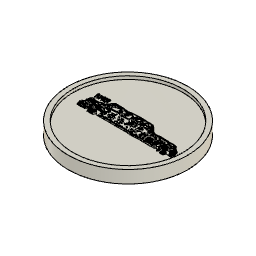
Pink Limo Cup Holder v2 (Autodesk Fusion 360 design; units mm, degrees)
Autodesk Fusion 360 part; units mm, degrees
(part 1 of 5)
sketch "Sketch1" plane through (0, 0, 0) normal (0, 0, 1) x (1, 0, 0)
  circle A0 centre (0, 0) radius 35
  circle A1 centre (0, 0) radius 38
  dimension "d1" = 70
  dimension "d2" = 3
  constraint coincident A0.centre A1.centre
  measures "d1" diameter of A0
extrude "Extrude1" add sketch "Sketch1" along normal blind 8
sketch "Sketch2" plane through (0, 0, 0) normal (0, 0, 1) x (1, 0, 0)
extrude "Extrude2" add sketch "Sketch1" along normal blind 4 contours A0
sketch "Sketch3" plane through (0, 0, 4) normal (0, 0, 1) x (-1, 0, 0)
  circle A0 centre (0, 0) radius 35
  spline S0 degree 3 poles (19.6297, -8.0291) (19.7741, -7.993) (19.7921, -7.8305) (19.7921, -6.2782) knots 0 0 0 0 1 1 1 1
  spline S1 degree 3 poles (19.7921, -6.2782) (19.7921, -5.0869) (19.765, -4.5815) (19.6928, -4.6176) knots 0 0 0 0 1 1 1 1
  spline S2 degree 3 poles (19.6928, -4.6176) (19.6387, -4.6537) (19.6206, -4.7349) (19.6477, -4.8071) knots 0 0 0 0 1 1 1 1
  spline S3 degree 3 poles (19.6477, -4.8071) (19.6748, -4.8703) (19.6387, -4.9876) (19.5665, -5.0598) knots 0 0 0 0 1 1 1 1
  spline S4 degree 3 poles (19.5665, -5.0598) (19.4762, -5.1501) (19.4311, -5.3757) (19.4311, -5.7367) knots 0 0 0 0 1 1 1 1
  spline S5 degree 3 poles (19.4311, -5.7367) (19.4311, -6.0436) (19.395, -6.2872) (19.3589, -6.2872) knots 0 0 0 0 1 1 1 1
  spline S6 degree 3 poles (19.3589, -6.2872) (19.1423, -6.2872) (18.9528, -6.0165) (18.9438, -5.6916) knots 0 0 0 0 1 1 1 1
  spline S7 degree 3 poles (18.9438, -5.6916) (18.9347, -5.4028) (18.9077, -5.3486) (18.7633, -5.3667) knots 0 0 0 0 1 1 1 1
  spline S8 degree 3 poles (18.7633, -5.3667) (18.5557, -5.4028) (18.4474, -5.2494) (18.4293, -4.8884) knots 0 0 0 0 1 1 1 1
  spline S9 degree 3 poles (18.4293, -4.8884) (18.4203, -4.6537) (18.4113, -4.6718) (18.3301, -5.0057) knots 0 0 0 0 1 1 1 1
  spline S10 degree 3 poles (18.3301, -5.0057) (18.2488, -5.3757) (18.2669, -5.4299) (18.6279, -5.9804) knots 0 0 0 0 1 1 1 1
  spline S11 degree 3 poles (18.6279, -5.9804) (18.9077, -6.4136) (18.9799, -6.5941) (18.9077, -6.6663) knots 0 0 0 0 1 1 1 1
  spline S12 degree 3 poles (18.9077, -6.6663) (18.8355, -6.7385) (18.7723, -6.7385) (18.673, -6.6573) knots 0 0 0 0 1 1 1 1
  spline S13 degree 3 poles (18.673, -6.6573) (18.5557, -6.558) (18.5376, -6.5851) (18.5467, -6.8468) knots 0 0 0 0 1 1 1 1
  spline S14 degree 3 poles (18.5467, -6.8468) (18.5557, -7.5327) (18.6189, -7.7312) (18.8716, -7.8576) knots 0 0 0 0 1 1 1 1
  spline S15 degree 3 poles (18.8716, -7.8576) (19.1965, -8.02) (19.4401, -8.0742) (19.6297, -8.0291) knots 0 0 0 0 1 1 1 1
  spline S16 degree 3 poles (19.034, -7.4966) (18.8806, -7.3432) (18.9438, -7.1356) (19.1965, -6.928) knots 0 0 0 0 1 1 1 1
  spline S17 degree 3 poles (19.1965, -6.928) (19.395, -6.7656) (19.5214, -6.8829) (19.5214, -7.2258) knots 0 0 0 0 1 1 1 1
  spline S18 degree 3 poles (19.5214, -7.2258) (19.5214, -7.6681) (19.3138, -7.7764) (19.034, -7.4966) knots 0 0 0 0 1 1 1 1
  spline S19 degree 3 poles (22.4635, -7.9298) (22.7794, -7.7222) (22.8696, -6.7295) (22.6711, -5.7187) knots 0 0 0 0 1 1 1 1
  spline S20 degree 3 poles (22.6711, -5.7187) (22.5808, -5.2855) (22.5357, -5.2133) (22.3732, -5.2313) knots 0 0 0 0 1 1 1 1
  spline S21 degree 3 poles (22.3732, -5.2313) (22.2198, -5.2494) (22.1747, -5.1862) (22.1386, -4.9425) knots 0 0 0 0 1 1 1 1
  spline S22 degree 3 poles (22.1386, -4.9425) (22.1115, -4.771) (22.0393, -4.6176) (21.9671, -4.5905) knots 0 0 0 0 1 1 1 1
  spline S23 degree 3 poles (21.9671, -4.5905) (21.8769, -4.5635) (21.8588, -4.6086) (21.8949, -4.762) knots 0 0 0 0 1 1 1 1
  spline S24 degree 3 poles (21.8949, -4.762) (21.922, -4.8793) (21.913, -5.0418) (21.8678, -5.114) knots 0 0 0 0 1 1 1 1
  spline S25 degree 3 poles (21.8678, -5.114) (21.8047, -5.2042) (21.7776, -5.2133) (21.7776, -5.1411) knots 0 0 0 0 1 1 1 1
  spline S26 degree 3 poles (21.7776, -5.1411) (21.7776, -5.0779) (21.7325, -5.0237) (21.6873, -5.0237) knots 0 0 0 0 1 1 1 1
  spline S27 degree 3 poles (21.6873, -5.0237) (21.6332, -5.0237) (21.5971, -5.2945) (21.5971, -5.6555) knots 0 0 0 0 1 1 1 1
  line L0 (21.5971, -5.6555) -> (21.5971, -6.2872)
  line L1 (21.5971, -6.2872) -> (21.8498, -6.2872)
  spline S28 degree 3 poles (21.8498, -6.2872) (21.9942, -6.2872) (22.1296, -6.2602) (22.1657, -6.2331) knots 0 0 0 0 1 1 1 1
  spline S29 degree 3 poles (22.1657, -6.2331) (22.2649, -6.1338) (22.1205, -5.9353) (21.9852, -5.9894) knots 0 0 0 0 1 1 1 1
  spline S30 degree 3 poles (21.9852, -5.9894) (21.8859, -6.0255) (21.8588, -5.9984) (21.8859, -5.8721) knots 0 0 0 0 1 1 1 1
  spline S31 degree 3 poles (21.8859, -5.8721) (21.931, -5.6194) (22.2559, -5.6555) (22.3281, -5.9262) knots 0 0 0 0 1 1 1 1
  spline S32 degree 3 poles (22.3281, -5.9262) (22.3642, -6.0526) (22.3913, -6.4497) (22.4003, -6.8107) knots 0 0 0 0 1 1 1 1
  spline S33 degree 3 poles (22.4003, -6.8107) (22.4093, -7.3973) (22.3913, -7.4695) (22.2469, -7.4424) knots 0 0 0 0 1 1 1 1
  spline S34 degree 3 poles (22.2469, -7.4424) (22.1657, -7.4244) (22.0754, -7.3161) (22.0664, -7.1897) knots 0 0 0 0 1 1 1 1
  spline S35 degree 3 poles (22.0664, -7.1897) (22.0483, -7.0634) (21.9852, -6.91) (21.931, -6.8468) knots 0 0 0 0 1 1 1 1
  spline S36 degree 3 poles (21.931, -6.8468) (21.8498, -6.7475) (21.8227, -6.7475) (21.7686, -6.8919) knots 0 0 0 0 1 1 1 1
  spline S37 degree 3 poles (21.7686, -6.8919) (21.7325, -6.9822) (21.6964, -7.1897) (21.6964, -7.3522) knots 0 0 0 0 1 1 1 1
  spline S38 degree 3 poles (21.6964, -7.3522) (21.6873, -7.8125) (22.1386, -8.1554) (22.4635, -7.9298) knots 0 0 0 0 1 1 1 1
  spline S39 degree 3 poles (2.1482, -7.8215) (3.2222, -7.7493) (4.6391, -7.5507) (5.9658, -7.271) knots 0 0 0 0 1 1 1 1
  spline S40 degree 3 poles (5.9658, -7.271) (7.0488, -7.0453) (7.7979, -7.0544) (8.9621, -7.298) knots 0 0 0 0 1 1 1 1
  spline S41 degree 3 poles (8.9621, -7.298) (9.9819, -7.5146) (10.0361, -7.5146) (13.2129, -7.5598) knots 0 0 0 0 1 1 1 1
  line L2 (13.2129, -7.5598) -> (15.3428, -7.5959)
  line L3 (15.3428, -7.5959) -> (15.7218, -7.3341)
  spline S42 degree 3 poles (15.7218, -7.3341) (16.2092, -6.9912) (16.8229, -6.1789) (17.229, -5.3035) knots 0 0 0 0 1 1 1 1
  spline S43 degree 3 poles (17.229, -5.3035) (17.7434, -4.2205) (17.8066, -4.1573) (18.6459, -3.9046) knots 0 0 0 0 1 1 1 1
  spline S44 degree 3 poles (18.6459, -3.9046) (19.0521, -3.7873) (19.7019, -3.6519) (20.0899, -3.6249) knots 0 0 0 0 1 1 1 1
  spline S45 degree 3 poles (20.0899, -3.6249) (20.5321, -3.5797) (20.857, -3.4985) (20.9924, -3.3992) knots 0 0 0 0 1 1 1 1
  spline S46 degree 3 poles (20.9924, -3.3992) (21.5339, -2.9751) (22.274, -2.8397) (22.9508, -3.0292) knots 0 0 0 0 1 1 1 1
  spline S47 degree 3 poles (22.9508, -3.0292) (23.0862, -3.0653) (23.3389, -3.0473) (23.5645, -2.966) knots 0 0 0 0 1 1 1 1
  spline S48 degree 3 poles (23.5645, -2.966) (23.9616, -2.8397) (23.9616, -2.8397) (24.2143, -3.1104) knots 0 0 0 0 1 1 1 1
  spline S49 degree 3 poles (24.2143, -3.1104) (24.3678, -3.2819) (24.5934, -3.4083) (24.801, -3.4534) knots 0 0 0 0 1 1 1 1
  spline S50 degree 3 poles (24.801, -3.4534) (25.3064, -3.5436) (26.1186, -3.4353) (26.2901, -3.2458) knots 0 0 0 0 1 1 1 1
  spline S51 degree 3 poles (26.2901, -3.2458) (26.6962, -2.8126) (27.1204, -0.8091) (26.9489, -0.1593) knots 0 0 0 0 1 1 1 1
  spline S52 degree 3 poles (26.9489, -0.1593) (26.8948, 0.0664) (26.9128, 0.2649) (27.0211, 0.6079) knots 0 0 0 0 1 1 1 1
  spline S53 degree 3 poles (27.0211, 0.6079) (27.1565, 1.005) (27.2197, 1.0681) (27.4363, 1.0952) knots 0 0 0 0 1 1 1 1
  spline S54 degree 3 poles (27.4363, 1.0952) (27.7612, 1.1313) (28.2936, 1.6367) (28.2305, 1.8443) knots 0 0 0 0 1 1 1 1
  spline S55 degree 3 poles (28.2305, 1.8443) (28.2034, 1.9255) (28.2395, 2.0428) (28.3207, 2.106) knots 0 0 0 0 1 1 1 1
  spline S56 degree 3 poles (28.3207, 2.106) (28.5102, 2.2594) (28.4922, 2.4038) (28.2756, 2.5392) knots 0 0 0 0 1 1 1 1
  spline S57 degree 3 poles (28.2756, 2.5392) (28.1673, 2.6024) (28.1131, 2.7017) (28.1492, 2.7558) knots 0 0 0 0 1 1 1 1
  spline S58 degree 3 poles (28.1492, 2.7558) (28.1853, 2.81) (28.1402, 2.9092) (28.05, 2.9724) knots 0 0 0 0 1 1 1 1
  spline S59 degree 3 poles (28.05, 2.9724) (27.9417, 3.0536) (27.8785, 3.2432) (27.8604, 3.6132) knots 0 0 0 0 1 1 1 1
  spline S60 degree 3 poles (27.8604, 3.6132) (27.8063, 4.281) (27.5355, 4.8767) (27.2106, 5.0121) knots 0 0 0 0 1 1 1 1
  spline S61 degree 3 poles (27.2106, 5.0121) (27.0482, 5.0843) (26.3081, 5.1113) (24.8912, 5.0933) knots 0 0 0 0 1 1 1 1
  spline S62 degree 3 poles (24.8912, 5.0933) (22.9328, 5.0662) (22.8064, 5.0572) (22.5718, 4.8767) knots 0 0 0 0 1 1 1 1
  spline S63 degree 3 poles (22.5718, 4.8767) (22.0213, 4.4525) (21.6061, 3.9832) (21.4978, 3.6583) knots 0 0 0 0 1 1 1 1
  spline S64 degree 3 poles (21.4978, 3.6583) (21.4437, 3.4778) (21.3715, 3.2612) (21.3444, 3.189) knots 0 0 0 0 1 1 1 1
  spline S65 degree 3 poles (21.3444, 3.189) (21.2902, 3.0175) (21.0375, 4.263) (21.0917, 4.4796) knots 0 0 0 0 1 1 1 1
  spline S66 degree 3 poles (21.0917, 4.4796) (21.1097, 4.5608) (21.0917, 4.6059) (21.0375, 4.5789) knots 0 0 0 0 1 1 1 1
  spline S67 degree 3 poles (21.0375, 4.5789) (20.9924, 4.5518) (20.9563, 4.5789) (20.9744, 4.642) knots 0 0 0 0 1 1 1 1
  spline S68 degree 3 poles (20.9744, 4.642) (21.0014, 4.9038) (20.9563, 5.003) (20.6404, 5.355) knots 0 0 0 0 1 1 1 1
  line L4 (20.6404, 5.355) -> (20.3156, 5.716)
  line L5 (20.3156, 5.716) -> (18.6279, 5.716)
  line L6 (18.6279, 5.716) -> (16.9402, 5.716)
  line L7 (16.9402, 5.716) -> (16.5251, 5.2828)
  spline S69 degree 3 poles (16.5251, 5.2828) (16.2724, 5.0301) (16.0558, 4.7052) (15.9836, 4.4796) knots 0 0 0 0 1 1 1 1
  line L8 (15.9836, 4.4796) -> (15.8662, 4.1005)
  line L9 (15.8662, 4.1005) -> (15.5504, 4.2901)
  spline S70 degree 3 poles (15.5504, 4.2901) (15.3789, 4.3984) (15.1442, 4.5698) (15.0269, 4.6691) knots 0 0 0 0 1 1 1 1
  spline S71 degree 3 poles (15.0269, 4.6691) (14.8284, 4.8496) (14.711, 4.8586) (12.9963, 4.8586) knots 0 0 0 0 1 1 1 1
  spline S72 degree 3 poles (12.9963, 4.8586) (11.9945, 4.8586) (10.5595, 4.8496) (9.8195, 4.8316) knots 0 0 0 0 1 1 1 1
  spline S73 degree 3 poles (9.8195, 4.8316) (9.0704, 4.8225) (6.1824, 4.8316) (3.3847, 4.8586) knots 0 0 0 0 1 1 1 1
  spline S74 degree 3 poles (3.3847, 4.8586) (0.0003, 4.8857) (-1.913, 4.8677) (-2.3462, 4.8045) knots 0 0 0 0 1 1 1 1
  spline S75 degree 3 poles (-2.3462, 4.8045) (-3.2036, 4.6691) (-3.2758, 4.6781) (-4.4851, 4.8496) knots 0 0 0 0 1 1 1 1
  spline S76 degree 3 poles (-4.4851, 4.8496) (-5.0537, 4.9308) (-5.8479, 5.0211) (-6.245, 5.0482) knots 0 0 0 0 1 1 1 1
  spline S77 degree 3 poles (-6.245, 5.0482) (-7.1295, 5.1113) (-11.8044, 4.9218) (-12.2647, 4.8045) knots 0 0 0 0 1 1 1 1
  spline S78 degree 3 poles (-12.2647, 4.8045) (-12.5084, 4.7413) (-12.6618, 4.7503) (-12.8062, 4.8225) knots 0 0 0 0 1 1 1 1
  spline S79 degree 3 poles (-12.8062, 4.8225) (-13.0228, 4.9399) (-14.891, 4.9579) (-18.9973, 4.8677) knots 0 0 0 0 1 1 1 1
  line L10 (-18.9973, 4.8677) -> (-21.1092, 4.8225)
  line L11 (-21.1092, 4.8225) -> (-21.3168, 4.5969)
  spline S80 degree 3 poles (-21.3168, 4.5969) (-21.4341, 4.4615) (-21.5875, 4.3623) (-21.6597, 4.3623) knots 0 0 0 0 1 1 1 1
  spline S81 degree 3 poles (-21.6597, 4.3623) (-21.7319, 4.3623) (-21.9756, 4.254) (-22.2102, 4.1276) knots 0 0 0 0 1 1 1 1
  spline S82 degree 3 poles (-22.2102, 4.1276) (-22.6344, 3.893) (-22.8059, 3.902) (-22.8149, 4.1637) knots 0 0 0 0 1 1 1 1
  spline S83 degree 3 poles (-22.8149, 4.1637) (-22.8239, 4.4525) (-23.3203, 5.2196) (-23.6181, 5.4272) knots 0 0 0 0 1 1 1 1
  spline S84 degree 3 poles (-23.6181, 5.4272) (-24.0062, 5.6889) (-24.1145, 5.6438) (-24.1145, 5.2377) knots 0 0 0 0 1 1 1 1
  spline S85 degree 3 poles (-24.1145, 5.2377) (-24.1145, 4.985) (-24.0784, 4.9128) (-23.9882, 4.9489) knots 0 0 0 0 1 1 1 1
  spline S86 degree 3 poles (-23.9882, 4.9489) (-23.8979, 4.985) (-23.9069, 4.9399) (-24.0152, 4.7684) knots 0 0 0 0 1 1 1 1
  spline S87 degree 3 poles (-24.0152, 4.7684) (-24.1687, 4.5337) (-24.0965, 4.4615) (-23.8889, 4.6601) knots 0 0 0 0 1 1 1 1
  spline S88 degree 3 poles (-23.8889, 4.6601) (-23.8257, 4.7142) (-23.8438, 4.6601) (-23.943, 4.5247) knots 0 0 0 0 1 1 1 1
  spline S89 degree 3 poles (-23.943, 4.5247) (-24.0423, 4.3713) (-24.1687, 4.2991) (-24.2499, 4.3262) knots 0 0 0 0 1 1 1 1
  spline S90 degree 3 poles (-24.2499, 4.3262) (-24.3582, 4.3623) (-24.3672, 4.3532) (-24.277, 4.263) knots 0 0 0 0 1 1 1 1
  spline S91 degree 3 poles (-24.277, 4.263) (-24.0152, 4.0013) (-24.2048, 2.9544) (-24.5838, 2.5392) knots 0 0 0 0 1 1 1 1
  spline S92 degree 3 poles (-24.5838, 2.5392) (-24.7914, 2.3046) (-24.8546, 2.3316) (-25.0531, 2.7378) knots 0 0 0 0 1 1 1 1
  line L12 (-25.0531, 2.7378) -> (-25.2246, 3.0988)
  line L13 (-25.2246, 3.0988) -> (-24.9899, 3.1078)
  spline S93 degree 3 poles (-24.9899, 3.1078) (-24.7643, 3.1258) (-24.7643, 3.1258) (-24.9538, 3.1619) knots 0 0 0 0 1 1 1 1
  spline S94 degree 3 poles (-24.9538, 3.1619) (-25.1253, 3.198) (-25.1524, 3.2432) (-25.1163, 3.4598) knots 0 0 0 0 1 1 1 1
  spline S95 degree 3 poles (-25.1163, 3.4598) (-25.0892, 3.6673) (-25.1073, 3.7034) (-25.2156, 3.6673) knots 0 0 0 0 1 1 1 1
  spline S96 degree 3 poles (-25.2156, 3.6673) (-25.3329, 3.6222) (-25.3419, 3.6403) (-25.2607, 3.7756) knots 0 0 0 0 1 1 1 1
  spline S97 degree 3 poles (-25.2607, 3.7756) (-25.1885, 3.92) (-25.2065, 3.9652) (-25.36, 4.0464) knots 0 0 0 0 1 1 1 1
  spline S98 degree 3 poles (-25.36, 4.0464) (-25.5856, 4.1547) (-25.6217, 4.3713) (-25.4322, 4.4345) knots 0 0 0 0 1 1 1 1
  spline S99 degree 3 poles (-25.4322, 4.4345) (-25.3419, 4.4615) (-25.3239, 4.4254) (-25.36, 4.281) knots 0 0 0 0 1 1 1 1
  spline S100 degree 3 poles (-25.36, 4.281) (-25.3961, 4.1186) (-25.387, 4.1005) (-25.2787, 4.1908) knots 0 0 0 0 1 1 1 1
  spline S101 degree 3 poles (-25.2787, 4.1908) (-25.1073, 4.3262) (-25.1163, 4.5879) (-25.3058, 4.7684) knots 0 0 0 0 1 1 1 1
  spline S102 degree 3 poles (-25.3058, 4.7684) (-25.4231, 4.8857) (-25.4322, 4.976) (-25.369, 5.1655) knots 0 0 0 0 1 1 1 1
  spline S103 degree 3 poles (-25.369, 5.1655) (-25.1795, 5.6889) (-25.2336, 5.716) (-26.461, 5.716) knots 0 0 0 0 1 1 1 1
  line L14 (-26.461, 5.716) -> (-27.5711, 5.716)
  line L15 (-27.5711, 5.716) -> (-27.887, 5.364)
  spline S104 degree 3 poles (-27.887, 5.364) (-28.0855, 5.1474) (-28.2299, 4.8677) (-28.266, 4.6601) knots 0 0 0 0 1 1 1 1
  spline S105 degree 3 poles (-28.266, 4.6601) (-28.3833, 3.9742) (-28.3653, 3.9922) (-28.9248, 4.0554) knots 0 0 0 0 1 1 1 1
  spline S106 degree 3 poles (-28.9248, 4.0554) (-29.2046, 4.0915) (-29.5385, 4.1637) (-29.6649, 4.2269) knots 0 0 0 0 1 1 1 1
  spline S107 degree 3 poles (-29.6649, 4.2269) (-29.7912, 4.2901) (-30.2786, 4.3623) (-30.7479, 4.3893) knots 0 0 0 0 1 1 1 1
  spline S108 degree 3 poles (-30.7479, 4.3893) (-31.4067, 4.4345) (-31.6594, 4.4164) (-31.8941, 4.3081) knots 0 0 0 0 1 1 1 1
  spline S109 degree 3 poles (-31.8941, 4.3081) (-32.3634, 4.0825) (-32.4265, 3.9561) (-32.237, 3.6042) knots 0 0 0 0 1 1 1 1
  spline S110 degree 3 poles (-32.237, 3.6042) (-32.0926, 3.3424) (-32.0836, 3.2612) (-32.1829, 3.0266) knots 0 0 0 0 1 1 1 1
  spline S111 degree 3 poles (-32.1829, 3.0266) (-32.2821, 2.8009) (-32.2731, 2.7107) (-32.1558, 2.4851) knots 0 0 0 0 1 1 1 1
  spline S112 degree 3 poles (-32.1558, 2.4851) (-32.0746, 2.3316) (-31.9753, 2.1782) (-31.9211, 2.1511) knots 0 0 0 0 1 1 1 1
  spline S113 degree 3 poles (-31.9211, 2.1511) (-31.7767, 2.0609) (-31.5601, 1.4833) (-31.5601, 1.1945) knots 0 0 0 0 1 1 1 1
  spline S114 degree 3 poles (-31.5601, 1.1945) (-31.5601, 0.0754) (-31.0006, -0.7008) (-30.0259, -0.9083) knots 0 0 0 0 1 1 1 1
  spline S115 degree 3 poles (-30.0259, -0.9083) (-29.8995, -0.9354) (-29.7281, -1.0708) (-29.6468, -1.2152) knots 0 0 0 0 1 1 1 1
  spline S116 degree 3 poles (-29.6468, -1.2152) (-29.5476, -1.3867) (-29.2949, -1.5672) (-28.9429, -1.7206) knots 0 0 0 0 1 1 1 1
  spline S117 degree 3 poles (-28.9429, -1.7206) (-28.5277, -1.9101) (-28.3653, -2.0365) (-28.275, -2.2531) knots 0 0 0 0 1 1 1 1
  spline S118 degree 3 poles (-28.275, -2.2531) (-28.2028, -2.4155) (-27.9592, -2.7224) (-27.7335, -2.948) knots 0 0 0 0 1 1 1 1
  line L16 (-27.7335, -2.948) -> (-27.3094, -3.3541)
  line L17 (-27.3094, -3.3541) -> (-26.0729, -3.3992)
  spline S119 degree 3 poles (-26.0729, -3.3992) (-25.3961, -3.4263) (-24.6741, -3.4173) (-24.4755, -3.3722) knots 0 0 0 0 1 1 1 1
  spline S120 degree 3 poles (-24.4755, -3.3722) (-23.8257, -3.2278) (-22.9683, -3.2548) (-22.4449, -3.4263) knots 0 0 0 0 1 1 1 1
  spline S121 degree 3 poles (-22.4449, -3.4263) (-22.0388, -3.5617) (-21.777, -3.5888) (-21.046, -3.5436) knots 0 0 0 0 1 1 1 1
  spline S122 degree 3 poles (-21.046, -3.5436) (-20.5496, -3.5166) (-19.3132, -3.5256) (-18.3024, -3.5797) knots 0 0 0 0 1 1 1 1
  spline S123 degree 3 poles (-18.3024, -3.5797) (-16.7952, -3.6429) (-16.3981, -3.6429) (-16.1815, -3.5346) knots 0 0 0 0 1 1 1 1
  spline S124 degree 3 poles (-16.1815, -3.5346) (-16.0281, -3.4714) (-15.5227, -3.3902) (-15.0624, -3.3631) knots 0 0 0 0 1 1 1 1
  spline S125 degree 3 poles (-15.0624, -3.3631) (-14.2863, -3.318) (-14.187, -3.327) (-13.7809, -3.5346) knots 0 0 0 0 1 1 1 1
  spline S126 degree 3 poles (-13.7809, -3.5346) (-13.5101, -3.67) (-13.1852, -3.7602) (-12.9506, -3.7602) knots 0 0 0 0 1 1 1 1
  spline S127 degree 3 poles (-12.9506, -3.7602) (-12.5715, -3.7602) (-12.5354, -3.7873) (-11.3893, -4.9515) knots 0 0 0 0 1 1 1 1
  spline S128 degree 3 poles (-11.3893, -4.9515) (-10.7395, -5.6104) (-9.855, -6.4677) (-9.4218, -6.8648) knots 0 0 0 0 1 1 1 1
  line L18 (-9.4218, -6.8648) -> (-8.6276, -7.5688)
  line L19 (-8.6276, -7.5688) -> (-7.9778, -7.632)
  spline S129 degree 3 poles (-7.9778, -7.632) (-7.6168, -7.6681) (-6.4526, -7.6951) (-5.3876, -7.6771) knots 0 0 0 0 1 1 1 1
  spline S130 degree 3 poles (-5.3876, -7.6771) (-4.3227, -7.6681) (-3.1404, -7.6861) (-2.7704, -7.7312) knots 0 0 0 0 1 1 1 1
  spline S131 degree 3 poles (-2.7704, -7.7312) (-1.8047, -7.8486) (0.975, -7.8937) (2.1482, -7.8215) knots 0 0 0 0 1 1 1 1
  spline S132 degree 3 poles (-0.7668, -7.4966) (-1.3715, -7.4515) (-1.5971, -7.3973) (-1.5971, -7.3161) knots 0 0 0 0 1 1 1 1
  spline S133 degree 3 poles (-1.5971, -7.3161) (-1.5971, -7.2439) (-1.6784, -7.1897) (-1.7686, -7.1897) knots 0 0 0 0 1 1 1 1
  spline S134 degree 3 poles (-1.7686, -7.1897) (-1.8679, -7.1897) (-2.0213, -7.1627) (-2.1116, -7.1266) knots 0 0 0 0 1 1 1 1
  spline S135 degree 3 poles (-2.1116, -7.1266) (-2.256, -7.0724) (-2.256, -7.0814) (-2.1477, -7.2168) knots 0 0 0 0 1 1 1 1
  spline S136 degree 3 poles (-2.1477, -7.2168) (-1.9581, -7.4515) (-2.0574, -7.4785) (-2.7162, -7.3612) knots 0 0 0 0 1 1 1 1
  spline S137 degree 3 poles (-2.7162, -7.3612) (-3.0411, -7.3071) (-3.4112, -7.28) (-3.5195, -7.3161) knots 0 0 0 0 1 1 1 1
  spline S138 degree 3 poles (-3.5195, -7.3161) (-3.6368, -7.3432) (-4.7559, -7.3702) (-6.0013, -7.3702) knots 0 0 0 0 1 1 1 1
  line L20 (-6.0013, -7.3702) -> (-8.2756, -7.3793)
  line L21 (-8.2756, -7.3793) -> (-9.3406, -6.4407)
  spline S139 degree 3 poles (-9.3406, -6.4407) (-9.9182, -5.9262) (-10.7846, -5.0779) (-11.2539, -4.5725) knots 0 0 0 0 1 1 1 1
  spline S140 degree 3 poles (-11.2539, -4.5725) (-12.1474, -3.6068) (-12.4542, -3.3992) (-13.0318, -3.3992) knots 0 0 0 0 1 1 1 1
  spline S141 degree 3 poles (-13.0318, -3.3992) (-13.3657, -3.3992) (-13.9614, -3.1195) (-13.9614, -2.966) knots 0 0 0 0 1 1 1 1
  spline S142 degree 3 poles (-13.9614, -2.966) (-13.9614, -2.9209) (-13.7899, -2.7946) (-13.5823, -2.6772) knots 0 0 0 0 1 1 1 1
  spline S143 degree 3 poles (-13.5823, -2.6772) (-12.9957, -2.3433) (-13.3026, -2.3704) (-14.2141, -2.7224) knots 0 0 0 0 1 1 1 1
  spline S144 degree 3 poles (-14.2141, -2.7224) (-15.1617, -3.0834) (-15.9469, -3.1556) (-15.9469, -2.8848) knots 0 0 0 0 1 1 1 1
  spline S145 degree 3 poles (-15.9469, -2.8848) (-15.9469, -2.7585) (-16.0191, -2.7946) (-16.2357, -3.0292) knots 0 0 0 0 1 1 1 1
  spline S146 degree 3 poles (-16.2357, -3.0292) (-16.5155, -3.327) (-16.5155, -3.327) (-17.1562, -3.2729) knots 0 0 0 0 1 1 1 1
  spline S147 degree 3 poles (-17.1562, -3.2729) (-17.5082, -3.2368) (-18.7537, -3.2097) (-19.9179, -3.2097) knots 0 0 0 0 1 1 1 1
  spline S148 degree 3 poles (-19.9179, -3.2097) (-21.0821, -3.2097) (-22.111, -3.1826) (-22.2012, -3.1556) knots 0 0 0 0 1 1 1 1
  spline S149 degree 3 poles (-22.2012, -3.1556) (-22.2824, -3.1375) (-22.3546, -3.0292) (-22.3546, -2.9299) knots 0 0 0 0 1 1 1 1
  spline S150 degree 3 poles (-22.3546, -2.9299) (-22.3546, -2.7494) (-22.3276, -2.7404) (-20.0984, -2.7855) knots 0 0 0 0 1 1 1 1
  spline S151 degree 3 poles (-20.0984, -2.7855) (-18.1309, -2.8216) (-17.8241, -2.8397) (-17.6797, -2.9841) knots 0 0 0 0 1 1 1 1
  spline S152 degree 3 poles (-17.6797, -2.9841) (-17.5263, -3.1104) (-17.4811, -3.1195) (-17.3819, -3.0112) knots 0 0 0 0 1 1 1 1
  spline S153 degree 3 poles (-17.3819, -3.0112) (-17.3097, -2.948) (-17.1021, -2.8668) (-16.9035, -2.8307) knots 0 0 0 0 1 1 1 1
  spline S154 degree 3 poles (-16.9035, -2.8307) (-16.344, -2.7404) (-16.1274, -2.5509) (-16.1274, -2.1357) knots 0 0 0 0 1 1 1 1
  spline S155 degree 3 poles (-16.1274, -2.1357) (-16.1274, -1.5491) (-16.8404, -0.8722) (-17.4721, -0.8722) knots 0 0 0 0 1 1 1 1
  spline S156 degree 3 poles (-17.4721, -0.8722) (-17.7158, -0.8722) (-17.7519, -0.8271) (-17.8421, -0.5022) knots 0 0 0 0 1 1 1 1
  spline S157 degree 3 poles (-17.8421, -0.5022) (-17.9234, -0.1954) (-17.9685, -0.1593) (-18.0768, -0.2405) knots 0 0 0 0 1 1 1 1
  spline S158 degree 3 poles (-18.0768, -0.2405) (-18.1761, -0.3307) (-18.2392, -0.3307) (-18.3475, -0.2315) knots 0 0 0 0 1 1 1 1
  spline S159 degree 3 poles (-18.3475, -0.2315) (-18.4739, -0.1322) (-18.51, -0.1322) (-18.6093, -0.2676) knots 0 0 0 0 1 1 1 1
  spline S160 degree 3 poles (-18.6093, -0.2676) (-18.6724, -0.3578) (-18.7807, -0.4029) (-18.871, -0.3668) knots 0 0 0 0 1 1 1 1
  spline S161 degree 3 poles (-18.871, -0.3668) (-18.9883, -0.3217) (-19.0154, -0.3668) (-19.0154, -0.5834) knots 0 0 0 0 1 1 1 1
  spline S162 degree 3 poles (-19.0154, -0.5834) (-19.0154, -0.8) (-19.0605, -0.8632) (-19.25, -0.9083) knots 0 0 0 0 1 1 1 1
  spline S163 degree 3 poles (-19.25, -0.9083) (-19.5388, -0.9805) (-19.6742, -0.8813) (-19.8998, -0.3939) knots 0 0 0 0 1 1 1 1
  spline S164 degree 3 poles (-19.8998, -0.3939) (-20.1886, 0.2288) (-20.2338, 0.7613) (-20.0262, 1.023) knots 0 0 0 0 1 1 1 1
  spline S165 degree 3 poles (-20.0262, 1.023) (-19.8728, 1.2125) (-19.8276, 1.2216) (-19.7013, 1.1223) knots 0 0 0 0 1 1 1 1
  spline S166 degree 3 poles (-19.7013, 1.1223) (-19.6201, 1.0501) (-19.5569, 0.8606) (-19.5569, 0.671) knots 0 0 0 0 1 1 1 1
  spline S167 degree 3 poles (-19.5569, 0.671) (-19.5569, 0.3913) (-19.2771, -0.2405) (-19.1508, -0.2405) knots 0 0 0 0 1 1 1 1
  spline S168 degree 3 poles (-19.1508, -0.2405) (-19.1327, -0.2405) (-18.9612, -0.1593) (-18.7807, -0.06) knots 0 0 0 0 1 1 1 1
  spline S169 degree 3 poles (-18.7807, -0.06) (-18.6002, 0.0483) (-18.3836, 0.1025) (-18.2844, 0.0754) knots 0 0 0 0 1 1 1 1
  spline S170 degree 3 poles (-18.2844, 0.0754) (-18.0587, 0.0032) (-18.0678, 0.1115) (-18.3475, 0.6891) knots 0 0 0 0 1 1 1 1
  spline S171 degree 3 poles (-18.3475, 0.6891) (-18.6363, 1.2667) (-18.6002, 1.5465) (-18.2031, 1.7631) knots 0 0 0 0 1 1 1 1
  line L22 (-18.2031, 1.7631) -> (-17.9324, 1.9165)
  line L23 (-17.9324, 1.9165) -> (-17.9324, 1.4743)
  spline S172 degree 3 poles (-17.9324, 1.4743) (-17.9324, 0.7252) (-17.6616, 0.1747) (-16.9396, -0.5293) knots 0 0 0 0 1 1 1 1
  spline S173 degree 3 poles (-16.9396, -0.5293) (-16.1815, -1.2693) (-15.8296, -1.4408) (-15.0715, -1.4408) knots 0 0 0 0 1 1 1 1
  spline S174 degree 3 poles (-15.0715, -1.4408) (-14.3585, -1.4318) (-14.0697, -1.3235) (-13.2665, -0.7188) knots 0 0 0 0 1 1 1 1
  spline S175 degree 3 poles (-13.2665, -0.7188) (-12.4452, -0.0961) (-12.2196, 0.3642) (-12.2105, 1.4291) knots 0 0 0 0 1 1 1 1
  spline S176 degree 3 poles (-12.2105, 1.4291) (-12.2015, 2.2143) (-12.3008, 2.476) (-12.8062, 3.0536) knots 0 0 0 0 1 1 1 1
  spline S177 degree 3 poles (-12.8062, 3.0536) (-12.9596, 3.2341) (-13.0589, 3.3966) (-13.0318, 3.4327) knots 0 0 0 0 1 1 1 1
  spline S178 degree 3 poles (-13.0318, 3.4327) (-13.0047, 3.4598) (-12.752, 3.4507) (-12.4903, 3.4237) knots 0 0 0 0 1 1 1 1
  line L24 (-12.4903, 3.4237) -> (-11.9939, 3.3605)
  line L25 (-11.9939, 3.3605) -> (-11.9217, 2.9363)
  spline S179 degree 3 poles (-11.9217, 2.9363) (-11.8856, 2.7017) (-11.8495, 1.1494) (-11.8405, -0.5112) knots 0 0 0 0 1 1 1 1
  spline S180 degree 3 poles (-11.8405, -0.5112) (-11.8405, -2.6321) (-11.8044, -3.5888) (-11.7322, -3.7241) knots 0 0 0 0 1 1 1 1
  spline S181 degree 3 poles (-11.7322, -3.7241) (-11.669, -3.8234) (-10.8748, -4.6447) (-9.9453, -5.5472) knots 0 0 0 0 1 1 1 1
  line L26 (-9.9453, -5.5472) -> (-8.2666, -7.1897)
  line L27 (-8.2666, -7.1897) -> (-7.5266, -7.1897)
  spline S182 degree 3 poles (-7.5266, -7.1897) (-7.1204, -7.1897) (-6.4797, -7.1446) (-6.1096, -7.0995) knots 0 0 0 0 1 1 1 1
  spline S183 degree 3 poles (-6.1096, -7.0995) (-4.8461, -6.937) (-4.6927, -6.6302) (-4.8371, -4.6176) knots 0 0 0 0 1 1 1 1
  spline S184 degree 3 poles (-4.8371, -4.6176) (-4.8913, -3.8776) (-4.9725, -2.9209) (-5.0266, -2.4967) knots 0 0 0 0 1 1 1 1
  spline S185 degree 3 poles (-5.0266, -2.4967) (-5.0718, -2.0726) (-5.1259, -0.5834) (-5.1349, 0.8245) knots 0 0 0 0 1 1 1 1
  line L28 (-5.1349, 0.8245) -> (-5.162, 3.3695)
  line L29 (-5.162, 3.3695) -> (-4.801, 3.3695)
  spline S186 degree 3 poles (-4.801, 3.3695) (-4.1512, 3.3695) (-3.7722, 3.2702) (-3.718, 3.0897) knots 0 0 0 0 1 1 1 1
  spline S187 degree 3 poles (-3.718, 3.0897) (-3.6368, 2.828) (-2.9509, 2.8461) (-2.8877, 3.1078) knots 0 0 0 0 1 1 1 1
  spline S188 degree 3 poles (-2.8877, 3.1078) (-2.8426, 3.2522) (-2.7794, 3.2883) (-2.5809, 3.2612) knots 0 0 0 0 1 1 1 1
  spline S189 degree 3 poles (-2.5809, 3.2612) (-2.4365, 3.2341) (-2.3191, 3.2522) (-2.3191, 3.2973) knots 0 0 0 0 1 1 1 1
  spline S190 degree 3 poles (-2.3191, 3.2973) (-2.3191, 3.3334) (-2.256, 3.3695) (-2.1838, 3.3695) knots 0 0 0 0 1 1 1 1
  spline S191 degree 3 poles (-2.1838, 3.3695) (-2.1116, 3.3695) (-2.0484, 3.3334) (-2.0484, 3.2883) knots 0 0 0 0 1 1 1 1
  spline S192 degree 3 poles (-2.0484, 3.2883) (-2.0484, 3.171) (-1.5249, 2.9814) (-1.3625, 3.0446) knots 0 0 0 0 1 1 1 1
  spline S193 degree 3 poles (-1.3625, 3.0446) (-1.2813, 3.0807) (-1.1549, 3.0536) (-1.0827, 2.9905) knots 0 0 0 0 1 1 1 1
  spline S194 degree 3 poles (-1.0827, 2.9905) (-0.9744, 2.9002) (-0.9293, 2.9092) (-0.8571, 3.0446) knots 0 0 0 0 1 1 1 1
  spline S195 degree 3 poles (-0.8571, 3.0446) (-0.7759, 3.198) (-0.7578, 3.198) (-0.5863, 3.0356) knots 0 0 0 0 1 1 1 1
  spline S196 degree 3 poles (-0.5863, 3.0356) (-0.3968, 2.8731) (-0.3968, 2.8731) (-0.4419, 3.0717) knots 0 0 0 0 1 1 1 1
  spline S197 degree 3 poles (-0.4419, 3.0717) (-0.5232, 3.3695) (-0.1351, 3.3515) (0.0635, 3.0536) knots 0 0 0 0 1 1 1 1
  spline S198 degree 3 poles (0.0635, 3.0536) (0.2169, 2.81) (0.4154, 2.7468) (0.3342, 2.9544) knots 0 0 0 0 1 1 1 1
  spline S199 degree 3 poles (0.3342, 2.9544) (0.271, 3.1258) (0.3884, 3.18) (0.632, 3.0897) knots 0 0 0 0 1 1 1 1
  spline S200 degree 3 poles (0.632, 3.0897) (0.7674, 3.0446) (0.8216, 2.9634) (0.7855, 2.8731) knots 0 0 0 0 1 1 1 1
  spline S201 degree 3 poles (0.7855, 2.8731) (0.7494, 2.8009) (0.7764, 2.7378) (0.8396, 2.7378) knots 0 0 0 0 1 1 1 1
  spline S202 degree 3 poles (0.8396, 2.7378) (0.8938, 2.7378) (0.966, 2.819) (0.993, 2.9183) knots 0 0 0 0 1 1 1 1
  spline S203 degree 3 poles (0.993, 2.9183) (1.0201, 3.0175) (1.1194, 3.0988) (1.2096, 3.0988) knots 0 0 0 0 1 1 1 1
  spline S204 degree 3 poles (1.2096, 3.0988) (1.3089, 3.0988) (1.4533, 3.1349) (1.5436, 3.18) knots 0 0 0 0 1 1 1 1
  spline S205 degree 3 poles (1.5436, 3.18) (2.1843, 3.4959) (3.0327, 3.5771) (3.5561, 3.3695) knots 0 0 0 0 1 1 1 1
  spline S206 degree 3 poles (3.5561, 3.3695) (3.7186, 3.2973) (3.863, 3.2973) (4.0345, 3.3695) knots 0 0 0 0 1 1 1 1
  spline S207 degree 3 poles (4.0345, 3.3695) (4.1698, 3.4146) (4.7655, 3.4598) (5.3611, 3.4598) knots 0 0 0 0 1 1 1 1
  spline S208 degree 3 poles (5.3611, 3.4598) (6.381, 3.4598) (6.8593, 3.3695) (6.751, 3.198) knots 0 0 0 0 1 1 1 1
  spline S209 degree 3 poles (6.751, 3.198) (6.7239, 3.1529) (6.769, 3.0897) (6.8503, 3.0627) knots 0 0 0 0 1 1 1 1
  spline S210 degree 3 poles (6.8503, 3.0627) (6.9586, 3.0266) (6.9766, 3.0536) (6.9315, 3.189) knots 0 0 0 0 1 1 1 1
  spline S211 degree 3 poles (6.9315, 3.189) (6.8773, 3.3515) (6.8864, 3.3515) (7.1571, 3.2251) knots 0 0 0 0 1 1 1 1
  spline S212 degree 3 poles (7.1571, 3.2251) (7.4369, 3.0807) (7.8791, 3.1168) (7.8791, 3.2793) knots 0 0 0 0 1 1 1 1
  spline S213 degree 3 poles (7.8791, 3.2793) (7.8791, 3.3334) (8.0416, 3.3695) (8.2311, 3.3695) knots 0 0 0 0 1 1 1 1
  line L30 (8.2311, 3.3695) -> (8.5831, 3.3695)
  line L31 (8.5831, 3.3695) -> (8.6372, 2.8009)
  spline S214 degree 3 poles (8.6372, 2.8009) (8.7726, 1.375) (8.9621, -1.4408) (8.9621, -1.9101) knots 0 0 0 0 1 1 1 1
  spline S215 degree 3 poles (8.9621, -1.9101) (8.9621, -2.4967) (9.1607, -3.9317) (9.4134, -5.1952) knots 0 0 0 0 1 1 1 1
  spline S216 degree 3 poles (9.4134, -5.1952) (9.6209, -6.197) (9.7563, -6.3775) (10.5415, -6.6573) knots 0 0 0 0 1 1 1 1
  spline S217 degree 3 poles (10.5415, -6.6573) (11.0108, -6.8287) (11.3267, -6.8558) (12.7887, -6.8829) knots 0 0 0 0 1 1 1 1
  spline S218 degree 3 poles (12.7887, -6.8829) (14.3771, -6.91) (14.5215, -6.9009) (14.7923, -6.7295) knots 0 0 0 0 1 1 1 1
  spline S219 degree 3 poles (14.7923, -6.7295) (15.1803, -6.4948) (15.8301, -5.4479) (16.1731, -4.4913) knots 0 0 0 0 1 1 1 1
  spline S220 degree 3 poles (16.1731, -4.4913) (16.4438, -3.7512) (16.4438, -3.7241) (16.3897, -2.4877) knots 0 0 0 0 1 1 1 1
  spline S221 degree 3 poles (16.3897, -2.4877) (16.3446, -1.4408) (16.3536, -1.2332) (16.4619, -1.2332) knots 0 0 0 0 1 1 1 1
  spline S222 degree 3 poles (16.4619, -1.2332) (16.5341, -1.2332) (16.9763, -1.3145) (17.4456, -1.4228) knots 0 0 0 0 1 1 1 1
  spline S223 degree 3 poles (17.4456, -1.4228) (18.7903, -1.7025) (19.2235, -1.6755) (20.3517, -1.2423) knots 0 0 0 0 1 1 1 1
  spline S224 degree 3 poles (20.3517, -1.2423) (20.8841, -1.0347) (21.4617, -0.7459) (21.6512, -0.5925) knots 0 0 0 0 1 1 1 1
  spline S225 degree 3 poles (21.6512, -0.5925) (21.8317, -0.4481) (22.1115, -0.2495) (22.274, -0.1502) knots 0 0 0 0 1 1 1 1
  spline S226 degree 3 poles (22.274, -0.1502) (22.4274, -0.051) (22.635, 0.1656) (22.7342, 0.3461) knots 0 0 0 0 1 1 1 1
  spline S227 degree 3 poles (22.7342, 0.3461) (22.8425, 0.5537) (23.0411, 0.7252) (23.3118, 0.8515) knots 0 0 0 0 1 1 1 1
  spline S228 degree 3 poles (23.3118, 0.8515) (23.5375, 0.9508) (23.9436, 1.2757) (24.2143, 1.5645) knots 0 0 0 0 1 1 1 1
  spline S229 degree 3 poles (24.2143, 1.5645) (24.6024, 1.9706) (24.828, 2.1241) (25.2612, 2.2775) knots 0 0 0 0 1 1 1 1
  spline S230 degree 3 poles (25.2612, 2.2775) (25.5681, 2.3858) (25.8298, 2.467) (25.8569, 2.467) knots 0 0 0 0 1 1 1 1
  spline S231 degree 3 poles (25.8569, 2.467) (25.884, 2.467) (25.9742, 2.2865) (26.0554, 2.0609) knots 0 0 0 0 1 1 1 1
  spline S232 degree 3 poles (26.0554, 2.0609) (26.1457, 1.8353) (26.3533, 1.5465) (26.5157, 1.4111) knots 0 0 0 0 1 1 1 1
  line L32 (26.5157, 1.4111) -> (26.8226, 1.1584)
  line L33 (26.8226, 1.1584) -> (26.6511, 0.662)
  spline S233 degree 3 poles (26.6511, 0.662) (26.5157, 0.2559) (26.3533, 0.0483) (25.7125, -0.5564) knots 0 0 0 0 1 1 1 1
  spline S234 degree 3 poles (25.7125, -0.5564) (25.2883, -0.9535) (24.7558, -1.504) (24.5212, -1.7747) knots 0 0 0 0 1 1 1 1
  spline S235 degree 3 poles (24.5212, -1.7747) (24.0248, -2.3523) (23.5555, -2.6772) (23.1945, -2.6772) knots 0 0 0 0 1 1 1 1
  spline S236 degree 3 poles (23.1945, -2.6772) (22.8967, -2.6772) (22.9508, -2.5058) (23.2487, -2.4877) knots 0 0 0 0 1 1 1 1
  spline S237 degree 3 poles (23.2487, -2.4877) (23.4021, -2.4787) (23.4111, -2.4697) (23.2848, -2.4336) knots 0 0 0 0 1 1 1 1
  spline S238 degree 3 poles (23.2848, -2.4336) (23.2035, -2.4155) (23.1494, -2.3614) (23.1674, -2.3253) knots 0 0 0 0 1 1 1 1
  spline S239 degree 3 poles (23.1674, -2.3253) (23.1945, -2.2892) (23.014, -2.3523) (22.7613, -2.4697) knots 0 0 0 0 1 1 1 1
  spline S240 degree 3 poles (22.7613, -2.4697) (22.4454, -2.6231) (22.2288, -2.6682) (22.0483, -2.6321) knots 0 0 0 0 1 1 1 1
  spline S241 degree 3 poles (22.0483, -2.6321) (21.7054, -2.5599) (21.1458, -2.6682) (21.2, -2.8036) knots 0 0 0 0 1 1 1 1
  spline S242 degree 3 poles (21.2, -2.8036) (21.2632, -2.9751) (20.6856, -3.2097) (20.1531, -3.2368) knots 0 0 0 0 1 1 1 1
  spline S243 degree 3 poles (20.1531, -3.2368) (19.738, -3.2548) (19.6567, -3.2278) (19.6297, -3.0924) knots 0 0 0 0 1 1 1 1
  spline S244 degree 3 poles (19.6297, -3.0924) (19.5845, -2.8938) (19.2867, -2.948) (19.3228, -3.1465) knots 0 0 0 0 1 1 1 1
  spline S245 degree 3 poles (19.3228, -3.1465) (19.3409, -3.2639) (19.1604, -3.3541) (18.5196, -3.5436) knots 0 0 0 0 1 1 1 1
  spline S246 degree 3 poles (18.5196, -3.5436) (17.7525, -3.7783) (17.6622, -3.8234) (17.4095, -4.1844) knots 0 0 0 0 1 1 1 1
  spline S247 degree 3 poles (17.4095, -4.1844) (17.2651, -4.401) (17.0485, -4.7981) (16.9402, -5.0779) knots 0 0 0 0 1 1 1 1
  spline S248 degree 3 poles (16.9402, -5.0779) (16.7146, -5.6104) (16.0828, -6.549) (15.7038, -6.91) knots 0 0 0 0 1 1 1 1
  spline S249 degree 3 poles (15.7038, -6.91) (15.3518, -7.2349) (14.4764, -7.3883) (13.5468, -7.28) knots 0 0 0 0 1 1 1 1
  spline S250 degree 3 poles (13.5468, -7.28) (13.1407, -7.2258) (12.157, -7.1897) (11.3808, -7.1897) knots 0 0 0 0 1 1 1 1
  spline S251 degree 3 poles (11.3808, -7.1897) (9.9639, -7.1897) (9.9639, -7.1897) (9.6661, -6.9461) knots 0 0 0 0 1 1 1 1
  spline S252 degree 3 poles (9.6661, -6.9461) (9.0794, -6.4497) (8.8719, -6.4046) (8.8719, -6.7656) knots 0 0 0 0 1 1 1 1
  spline S253 degree 3 poles (8.8719, -6.7656) (8.8719, -6.8919) (8.8358, -6.919) (8.7094, -6.8648) knots 0 0 0 0 1 1 1 1
  spline S254 degree 3 poles (8.7094, -6.8648) (8.3304, -6.7024) (6.7961, -6.7204) (5.9568, -6.91) knots 0 0 0 0 1 1 1 1
  spline S255 degree 3 poles (5.9568, -6.91) (3.6283, -7.4154) (1.1826, -7.632) (-0.7668, -7.4966) knots 0 0 0 0 1 1 1 1
  line L34 (-8.3388, -6.8739) -> (-8.5915, -6.6392)
  line L35 (-8.5915, -6.6392) -> (-8.2125, -6.8378)
  spline S256 degree 3 poles (-8.2125, -6.8378) (-7.7973, -7.0363) (-7.7432, -7.0995) (-7.9507, -7.0995) knots 0 0 0 0 1 1 1 1
  spline S257 degree 3 poles (-7.9507, -7.0995) (-8.0229, -7.0995) (-8.2034, -7.0002) (-8.3388, -6.8739) knots 0 0 0 0 1 1 1 1
  spline S258 degree 3 poles (-5.866, -6.7836) (-5.3606, -6.567) (-5.2613, -6.3053) (-5.3245, -5.3125) knots 0 0 0 0 1 1 1 1
  spline S259 degree 3 poles (-5.3245, -5.3125) (-5.4418, -3.5075) (-5.6313, -3.3) (-7.2107, -3.2909) knots 0 0 0 0 1 1 1 1
  spline S260 degree 3 poles (-7.2107, -3.2909) (-8.0049, -3.2909) (-8.1673, -3.2639) (-8.3298, -3.1104) knots 0 0 0 0 1 1 1 1
  spline S261 degree 3 poles (-8.3298, -3.1104) (-8.6186, -2.8487) (-9.6384, -2.6953) (-10.0175, -2.8577) knots 0 0 0 0 1 1 1 1
  spline S262 degree 3 poles (-10.0175, -2.8577) (-10.1799, -2.9209) (-10.5138, -2.9841) (-10.7575, -2.9841) knots 0 0 0 0 1 1 1 1
  spline S263 degree 3 poles (-10.7575, -2.9841) (-11.1636, -2.9931) (-11.2088, -3.0112) (-11.2358, -3.2097) knots 0 0 0 0 1 1 1 1
  spline S264 degree 3 poles (-11.2358, -3.2097) (-11.281, -3.4985) (-11.1095, -3.8054) (-10.8387, -3.9317) knots 0 0 0 0 1 1 1 1
  spline S265 degree 3 poles (-10.8387, -3.9317) (-10.7214, -3.9859) (-10.6221, -4.0851) (-10.6221, -4.1573) knots 0 0 0 0 1 1 1 1
  spline S266 degree 3 poles (-10.6221, -4.1573) (-10.6221, -4.3108) (-10.1167, -4.753) (-9.9362, -4.753) knots 0 0 0 0 1 1 1 1
  spline S267 degree 3 poles (-9.9362, -4.753) (-9.864, -4.753) (-9.8099, -4.8342) (-9.8099, -4.9425) knots 0 0 0 0 1 1 1 1
  spline S268 degree 3 poles (-9.8099, -4.9425) (-9.8099, -5.1772) (-9.6655, -5.4479) (-9.3677, -5.7909) knots 0 0 0 0 1 1 1 1
  spline S269 degree 3 poles (-9.3677, -5.7909) (-8.9164, -6.2963) (-9.476, -5.8089) (-10.5048, -4.7981) knots 0 0 0 0 1 1 1 1
  spline S270 degree 3 poles (-10.5048, -4.7981) (-11.1005, -4.2205) (-11.5607, -3.6971) (-11.6059, -3.5346) knots 0 0 0 0 1 1 1 1
  spline S271 degree 3 poles (-11.6059, -3.5346) (-11.651, -3.3902) (-11.7051, -1.7928) (-11.7232, 0.0032) knots 0 0 0 0 1 1 1 1
  line L36 (-11.7232, 0.0032) -> (-11.7593, 3.2702)
  line L37 (-11.7593, 3.2702) -> (-11.3261, 3.3785)
  spline S272 degree 3 poles (-11.3261, 3.3785) (-11.0824, 3.4327) (-10.8207, 3.4507) (-10.7485, 3.4237) knots 0 0 0 0 1 1 1 1
  spline S273 degree 3 poles (-10.7485, 3.4237) (-10.6673, 3.3876) (-10.5409, 3.4146) (-10.4777, 3.4688) knots 0 0 0 0 1 1 1 1
  spline S274 degree 3 poles (-10.4777, 3.4688) (-10.3785, 3.55) (-10.3514, 3.541) (-10.3514, 3.4237) knots 0 0 0 0 1 1 1 1
  spline S275 degree 3 poles (-10.3514, 3.4237) (-10.3514, 3.2702) (-10.1258, 3.2251) (-10.0355, 3.3695) knots 0 0 0 0 1 1 1 1
  spline S276 degree 3 poles (-10.0355, 3.3695) (-10.0084, 3.4237) (-9.9001, 3.4146) (-9.7648, 3.3515) knots 0 0 0 0 1 1 1 1
  spline S277 degree 3 poles (-9.7648, 3.3515) (-9.5933, 3.2702) (-9.485, 3.2793) (-9.2955, 3.3695) knots 0 0 0 0 1 1 1 1
  spline S278 degree 3 poles (-9.2955, 3.3695) (-9.1511, 3.4417) (-8.781, 3.4959) (-8.4561, 3.5049) knots 0 0 0 0 1 1 1 1
  spline S279 degree 3 poles (-8.4561, 3.5049) (-8.1312, 3.5049) (-7.5988, 3.541) (-7.2739, 3.5861) knots 0 0 0 0 1 1 1 1
  spline S280 degree 3 poles (-7.2739, 3.5861) (-6.6692, 3.6673) (-5.6133, 3.5951) (-5.4057, 3.4688) knots 0 0 0 0 1 1 1 1
  spline S281 degree 3 poles (-5.4057, 3.4688) (-5.3245, 3.4146) (-5.2884, 2.837) (-5.2884, 1.1042) knots 0 0 0 0 1 1 1 1
  spline S282 degree 3 poles (-5.2884, 1.1042) (-5.2884, -0.1593) (-5.2523, -1.5762) (-5.2071, -2.0455) knots 0 0 0 0 1 1 1 1
  spline S283 degree 3 poles (-5.2071, -2.0455) (-5.162, -2.5148) (-5.0808, -3.6158) (-5.0176, -4.4822) knots 0 0 0 0 1 1 1 1
  spline S284 degree 3 poles (-5.0176, -4.4822) (-4.9183, -5.8901) (-4.9274, -6.0977) (-5.0537, -6.4046) knots 0 0 0 0 1 1 1 1
  spline S285 degree 3 poles (-5.0537, -6.4046) (-5.2071, -6.7656) (-5.4418, -6.91) (-5.884, -6.91) knots 0 0 0 0 1 1 1 1
  line L38 (-5.884, -6.91) -> (-6.1548, -6.91)
  line L39 (-6.1548, -6.91) -> (-5.866, -6.7836)
  spline S286 degree 3 poles (11.805, -6.7114) (11.0469, -6.6843) (10.713, -6.6392) (10.4061, -6.4948) knots 0 0 0 0 1 1 1 1
  spline S287 degree 3 poles (10.4061, -6.4948) (9.7383, -6.197) (9.7022, -6.1067) (9.4043, -4.3739) knots 0 0 0 0 1 1 1 1
  spline S288 degree 3 poles (9.4043, -4.3739) (9.1155, -2.6592) (9.0975, -2.3343) (9.2419, -1.865) knots 0 0 0 0 1 1 1 1
  spline S289 degree 3 poles (9.2419, -1.865) (9.287, -1.6935) (9.3682, -1.1971) (9.4134, -0.7639) knots 0 0 0 0 1 1 1 1
  spline S290 degree 3 poles (9.4134, -0.7639) (9.4946, 0.1025) (9.4134, 0.644) (9.1426, 1.032) knots 0 0 0 0 1 1 1 1
  spline S291 degree 3 poles (9.1426, 1.032) (8.9441, 1.3028) (8.7455, 2.467) (8.7997, 3.0627) knots 0 0 0 0 1 1 1 1
  line L40 (8.7997, 3.0627) -> (8.8267, 3.4146)
  line L41 (8.8267, 3.4146) -> (11.1913, 3.4417)
  spline S292 degree 3 poles (11.1913, 3.4417) (13.4295, 3.4688) (13.5649, 3.4598) (13.5649, 3.3063) knots 0 0 0 0 1 1 1 1
  spline S293 degree 3 poles (13.5649, 3.3063) (13.5649, 3.2161) (13.6822, 2.9002) (13.8266, 2.6024) knots 0 0 0 0 1 1 1 1
  spline S294 degree 3 poles (13.8266, 2.6024) (14.0522, 2.1511) (14.2959, 1.4923) (14.5305, 0.7342) knots 0 0 0 0 1 1 1 1
  spline S295 degree 3 poles (14.5305, 0.7342) (14.5666, 0.6259) (14.5305, 0.5718) (14.4313, 0.5718) knots 0 0 0 0 1 1 1 1
  spline S296 degree 3 poles (14.4313, 0.5718) (14.2688, 0.5718) (14.2327, 0.3461) (14.3771, 0.2559) knots 0 0 0 0 1 1 1 1
  spline S297 degree 3 poles (14.3771, 0.2559) (14.4313, 0.2198) (14.5396, 0.2469) (14.6118, 0.31) knots 0 0 0 0 1 1 1 1
  spline S298 degree 3 poles (14.6118, 0.31) (14.7291, 0.4093) (14.7652, 0.4003) (14.8284, 0.301) knots 0 0 0 0 1 1 1 1
  spline S299 degree 3 poles (14.8284, 0.301) (15.0901, -0.1683) (15.3879, -0.5022) (15.7579, -0.782) knots 0 0 0 0 1 1 1 1
  line L42 (15.7579, -0.782) -> (16.1821, -1.0979)
  line L43 (16.1821, -1.0979) -> (16.1821, -1.7838)
  spline S300 degree 3 poles (16.1821, -1.7838) (16.1821, -2.1538) (16.2272, -2.6863) (16.2724, -2.966) knots 0 0 0 0 1 1 1 1
  spline S301 degree 3 poles (16.2724, -2.966) (16.3626, -3.4263) (16.3446, -3.5436) (16.0919, -4.2566) knots 0 0 0 0 1 1 1 1
  spline S302 degree 3 poles (16.0919, -4.2566) (15.6226, -5.6284) (14.9186, -6.6843) (14.4403, -6.7565) knots 0 0 0 0 1 1 1 1
  spline S303 degree 3 poles (14.4403, -6.7565) (14.332, -6.7746) (13.9168, -6.7746) (13.5197, -6.7656) knots 0 0 0 0 1 1 1 1
  spline S304 degree 3 poles (13.5197, -6.7656) (13.1226, -6.7475) (12.3465, -6.7295) (11.805, -6.7114) knots 0 0 0 0 1 1 1 1
  spline S305 degree 3 poles (-8.8803, -5.7277) (-9.1962, -5.3847) (-9.3767, -5.0689) (-9.2955, -4.9876) knots 0 0 0 0 1 1 1 1
  spline S306 degree 3 poles (-9.2955, -4.9876) (-9.2684, -4.9606) (-9.0879, -4.9335) (-8.9074, -4.9335) knots 0 0 0 0 1 1 1 1
  spline S307 degree 3 poles (-8.9074, -4.9335) (-8.6276, -4.9335) (-8.5283, -4.8793) (-8.3388, -4.6357) knots 0 0 0 0 1 1 1 1
  spline S308 degree 3 poles (-8.3388, -4.6357) (-8.2125, -4.4642) (-8.0951, -4.2115) (-8.0771, -4.0671) knots 0 0 0 0 1 1 1 1
  line L44 (-8.0771, -4.0671) -> (-8.05, -3.8054)
  line L45 (-8.05, -3.8054) -> (-7.2829, -3.7783)
  spline S309 degree 3 poles (-7.2829, -3.7783) (-6.0104, -3.7332) (-5.9833, -3.7602) (-5.884, -4.9154) knots 0 0 0 0 1 1 1 1
  line L46 (-5.884, -4.9154) -> (-5.8118, -5.6555)
  line L47 (-5.8118, -5.6555) -> (-6.0555, -5.6555)
  spline S310 degree 3 poles (-6.0555, -5.6555) (-6.2631, -5.6555) (-6.2901, -5.6194) (-6.2901, -5.3306) knots 0 0 0 0 1 1 1 1
  spline S311 degree 3 poles (-6.2901, -5.3306) (-6.2901, -5.0237) (-6.2992, -5.0147) (-6.5519, -5.0689) knots 0 0 0 0 1 1 1 1
  spline S312 degree 3 poles (-6.5519, -5.0689) (-6.7775, -5.114) (-6.8226, -5.0869) (-6.9219, -4.8432) knots 0 0 0 0 1 1 1 1
  spline S313 degree 3 poles (-6.9219, -4.8432) (-7.0392, -4.5635) (-7.1926, -4.4732) (-7.1926, -4.6898) knots 0 0 0 0 1 1 1 1
  spline S314 degree 3 poles (-7.1926, -4.6898) (-7.1926, -4.753) (-7.2468, -4.8793) (-7.31, -4.9696) knots 0 0 0 0 1 1 1 1
  spline S315 degree 3 poles (-7.31, -4.9696) (-7.4092, -5.105) (-7.4634, -5.123) (-7.6258, -5.0328) knots 0 0 0 0 1 1 1 1
  spline S316 degree 3 poles (-7.6258, -5.0328) (-7.8063, -4.9335) (-7.8244, -4.9515) (-7.8244, -5.1501) knots 0 0 0 0 1 1 1 1
  spline S317 degree 3 poles (-7.8244, -5.1501) (-7.8244, -5.5111) (-7.9237, -5.6555) (-8.1583, -5.6555) knots 0 0 0 0 1 1 1 1
  spline S318 degree 3 poles (-8.1583, -5.6555) (-8.3027, -5.6555) (-8.402, -5.7187) (-8.4291, -5.836) knots 0 0 0 0 1 1 1 1
  spline S319 degree 3 poles (-8.4291, -5.836) (-8.4922, -6.0797) (-8.5554, -6.0616) (-8.8803, -5.7277) knots 0 0 0 0 1 1 1 1
  spline S320 degree 3 poles (-10.0626, -4.5093) (-10.4326, -4.3198) (-10.5499, -4.1212) (-10.2702, -4.1212) knots 0 0 0 0 1 1 1 1
  spline S321 degree 3 poles (-10.2702, -4.1212) (-9.9272, -4.1212) (-9.7738, -3.5075) (-10.0445, -3.2097) knots 0 0 0 0 1 1 1 1
  spline S322 degree 3 poles (-10.0445, -3.2097) (-10.1799, -3.0563) (-10.1709, -3.0382) (-9.9543, -2.9841) knots 0 0 0 0 1 1 1 1
  spline S323 degree 3 poles (-9.9543, -2.9841) (-9.6835, -2.9209) (-8.9345, -3.0021) (-8.5915, -3.1285) knots 0 0 0 0 1 1 1 1
  spline S324 degree 3 poles (-8.5915, -3.1285) (-8.2847, -3.2458) (-8.1312, -3.8234) (-8.3117, -4.2386) knots 0 0 0 0 1 1 1 1
  spline S325 degree 3 poles (-8.3117, -4.2386) (-8.5013, -4.7079) (-8.7359, -4.8252) (-9.2774, -4.744) knots 0 0 0 0 1 1 1 1
  spline S326 degree 3 poles (-9.2774, -4.744) (-9.5301, -4.7079) (-9.8821, -4.5996) (-10.0626, -4.5093) knots 0 0 0 0 1 1 1 1
  spline S327 degree 3 poles (-10.6221, -3.8054) (-10.8929, -3.67) (-10.938, -3.5436) (-10.8387, -3.2729) knots 0 0 0 0 1 1 1 1
  spline S328 degree 3 poles (-10.8387, -3.2729) (-10.7756, -3.1014) (-10.5319, -3.1917) (-10.5319, -3.3992) knots 0 0 0 0 1 1 1 1
  spline S329 degree 3 poles (-10.5319, -3.3992) (-10.5319, -3.5978) (-10.3153, -3.688) (-10.1799, -3.5527) knots 0 0 0 0 1 1 1 1
  spline S330 degree 3 poles (-10.1799, -3.5527) (-10.0626, -3.4353) (-10.0445, -3.5617) (-10.1348, -3.7963) knots 0 0 0 0 1 1 1 1
  spline S331 degree 3 poles (-10.1348, -3.7963) (-10.207, -3.9768) (-10.2882, -3.9768) (-10.6221, -3.8054) knots 0 0 0 0 1 1 1 1
  spline S332 degree 3 poles (24.458, -2.8397) (24.3046, -2.6321) (24.2956, -2.587) (24.4129, -2.4245) knots 0 0 0 0 1 1 1 1
  spline S333 degree 3 poles (24.4129, -2.4245) (24.6927, -2.0184) (25.4056, -1.3235) (25.4869, -1.3686) knots 0 0 0 0 1 1 1 1
  spline S334 degree 3 poles (25.4869, -1.3686) (25.532, -1.4047) (25.5681, -1.7025) (25.5681, -2.0545) knots 0 0 0 0 1 1 1 1
  spline S335 degree 3 poles (25.5681, -2.0545) (25.5681, -2.4065) (25.6042, -2.6772) (25.6583, -2.6772) knots 0 0 0 0 1 1 1 1
  spline S336 degree 3 poles (25.6583, -2.6772) (25.7035, -2.6772) (25.7486, -2.596) (25.7486, -2.4967) knots 0 0 0 0 1 1 1 1
  spline S337 degree 3 poles (25.7486, -2.4967) (25.7486, -2.3975) (25.7847, -2.3162) (25.8298, -2.3162) knots 0 0 0 0 1 1 1 1
  spline S338 degree 3 poles (25.8298, -2.3162) (25.9471, -2.3162) (26.0193, -1.9643) (25.9201, -1.9011) knots 0 0 0 0 1 1 1 1
  spline S339 degree 3 poles (25.9201, -1.9011) (25.8659, -1.874) (25.8749, -1.7928) (25.9381, -1.7116) knots 0 0 0 0 1 1 1 1
  spline S340 degree 3 poles (25.9381, -1.7116) (26.0284, -1.6033) (26.0284, -1.5672) (25.9201, -1.495) knots 0 0 0 0 1 1 1 1
  spline S341 degree 3 poles (25.9201, -1.495) (25.8118, -1.4318) (25.8118, -1.4047) (25.9201, -1.3325) knots 0 0 0 0 1 1 1 1
  spline S342 degree 3 poles (25.9201, -1.3325) (26.0013, -1.2784) (26.0103, -1.2332) (25.9381, -1.1971) knots 0 0 0 0 1 1 1 1
  spline S343 degree 3 poles (25.9381, -1.1971) (25.8298, -1.1249) (25.9381, -0.8813) (26.2359, -0.5383) knots 0 0 0 0 1 1 1 1
  spline S344 degree 3 poles (26.2359, -0.5383) (26.4977, -0.2315) (26.5879, -0.2856) (26.5157, -0.7098) knots 0 0 0 0 1 1 1 1
  spline S345 degree 3 poles (26.5157, -0.7098) (26.4796, -0.9174) (26.4345, -1.3145) (26.4255, -1.5852) knots 0 0 0 0 1 1 1 1
  spline S346 degree 3 poles (26.4255, -1.5852) (26.3984, -2.1267) (26.1547, -2.948) (25.9832, -3.0653) knots 0 0 0 0 1 1 1 1
  spline S347 degree 3 poles (25.9832, -3.0653) (25.9291, -3.1014) (25.6042, -3.1195) (25.2612, -3.1104) knots 0 0 0 0 1 1 1 1
  spline S348 degree 3 poles (25.2612, -3.1104) (24.7107, -3.0834) (24.6205, -3.0563) (24.458, -2.8397) knots 0 0 0 0 1 1 1 1
  spline S349 degree 3 poles (-27.5169, -2.6953) (-27.6974, -2.5238) (-27.896, -2.2621) (-27.9411, -2.1177) knots 0 0 0 0 1 1 1 1
  spline S350 degree 3 poles (-27.9411, -2.1177) (-28.0314, -1.865) (-28.0314, -1.856) (-27.7426, -1.9011) knots 0 0 0 0 1 1 1 1
  spline S351 degree 3 poles (-27.7426, -1.9011) (-27.5801, -1.9282) (-26.9303, -1.9733) (-26.2805, -2.0004) knots 0 0 0 0 1 1 1 1
  spline S352 degree 3 poles (-26.2805, -2.0004) (-25.378, -2.0365) (-24.9899, -2.0184) (-24.6109, -1.9101) knots 0 0 0 0 1 1 1 1
  spline S353 degree 3 poles (-24.6109, -1.9101) (-23.9972, -1.7477) (-23.8889, -1.7386) (-23.8889, -1.9011) knots 0 0 0 0 1 1 1 1
  spline S354 degree 3 poles (-23.8889, -1.9011) (-23.8889, -2.1628) (-23.6362, -2.1267) (-23.5369, -1.856) knots 0 0 0 0 1 1 1 1
  spline S355 degree 3 poles (-23.5369, -1.856) (-23.4376, -1.5672) (-23.212, -1.4859) (-23.3023, -1.7747) knots 0 0 0 0 1 1 1 1
  spline S356 degree 3 poles (-23.3023, -1.7747) (-23.3654, -1.9823) (-23.1398, -2.4606) (-22.8961, -2.6141) knots 0 0 0 0 1 1 1 1
  spline S357 degree 3 poles (-22.8961, -2.6141) (-22.5893, -2.7946) (-22.6705, -2.957) (-23.0044, -2.8397) knots 0 0 0 0 1 1 1 1
  spline S358 degree 3 poles (-23.0044, -2.8397) (-23.221, -2.7585) (-23.3023, -2.7675) (-23.3293, -2.8397) knots 0 0 0 0 1 1 1 1
  spline S359 degree 3 poles (-23.3293, -2.8397) (-23.3474, -2.9119) (-23.5098, -2.9299) (-23.8347, -2.8938) knots 0 0 0 0 1 1 1 1
  spline S360 degree 3 poles (-23.8347, -2.8938) (-24.2228, -2.8487) (-24.3221, -2.8668) (-24.3672, -2.9841) knots 0 0 0 0 1 1 1 1
  spline S361 degree 3 poles (-24.3672, -2.9841) (-24.4214, -3.1104) (-24.5838, -3.1195) (-25.8022, -3.0743) knots 0 0 0 0 1 1 1 1
  line L48 (-25.8022, -3.0743) -> (-27.183, -3.0202)
  line L49 (-27.183, -3.0202) -> (-27.5169, -2.6953)
  spline S362 degree 3 poles (-20.2789, -2.587) (-20.2789, -2.5419) (-20.2338, -2.4967) (-20.1796, -2.4967) knots 0 0 0 0 1 1 1 1
  spline S363 degree 3 poles (-20.1796, -2.4967) (-20.1345, -2.4967) (-20.1164, -2.5419) (-20.1435, -2.587) knots 0 0 0 0 1 1 1 1
  spline S364 degree 3 poles (-20.1435, -2.587) (-20.1706, -2.6411) (-20.2157, -2.6772) (-20.2428, -2.6772) knots 0 0 0 0 1 1 1 1
  spline S365 degree 3 poles (-20.2428, -2.6772) (-20.2608, -2.6772) (-20.2789, -2.6411) (-20.2789, -2.587) knots 0 0 0 0 1 1 1 1
  spline S366 degree 3 poles (-22.3546, -2.5509) (-22.3546, -2.5238) (-22.3185, -2.4787) (-22.2644, -2.4516) knots 0 0 0 0 1 1 1 1
  spline S367 degree 3 poles (-22.2644, -2.4516) (-22.2193, -2.4245) (-22.1741, -2.4426) (-22.1741, -2.4877) knots 0 0 0 0 1 1 1 1
  spline S368 degree 3 poles (-22.1741, -2.4877) (-22.1741, -2.5419) (-22.2193, -2.587) (-22.2644, -2.587) knots 0 0 0 0 1 1 1 1
  spline S369 degree 3 poles (-22.2644, -2.587) (-22.3185, -2.587) (-22.3546, -2.5689) (-22.3546, -2.5509) knots 0 0 0 0 1 1 1 1
  spline S370 degree 3 poles (-22.6254, -2.5509) (-22.6254, -2.5238) (-22.5893, -2.4787) (-22.5351, -2.4516) knots 0 0 0 0 1 1 1 1